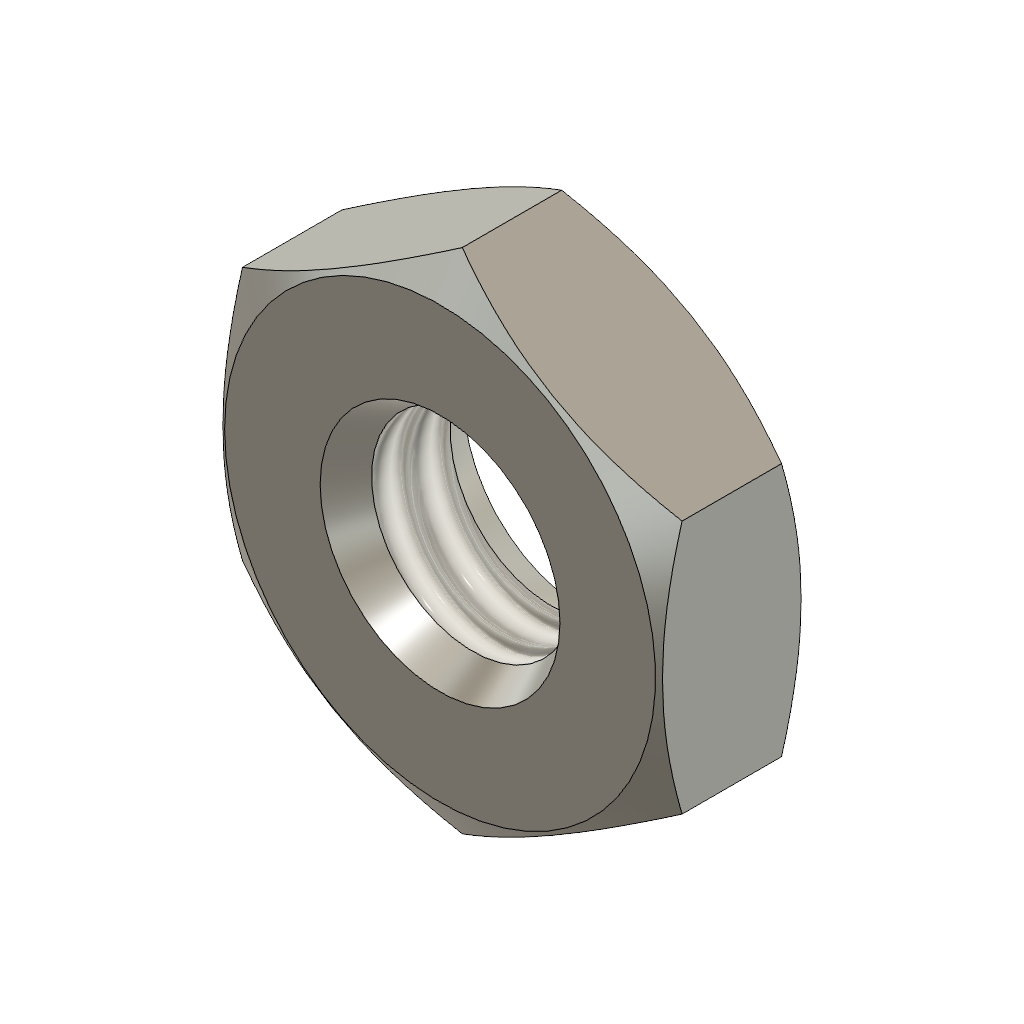
pencarriage (Autodesk Fusion 360 archive; units mm, degrees)
design "Hexagon Thin Nut ISO 4035 - M3 Steel 6 Plain"
description: Hexagon Thin Nut ISO 4035 - M3
part number: ISO 4035 - M3 Steel 6 Plain
Autodesk Fusion 360 part; units mm, degrees
sketch "Sketch1" plane through (0, 0, 0) normal (0, 1, 0) x (1, 0, 0)
  line L0 (0, 0) -> (0, -1.8)
  line L1 (-1.5, 0) -> (-2.695, 0)
  line L2 (-2.695, 0) -> (-3.1763, -0.2778)
  line L3 (-3.1763, -0.2778) -> (-3.1763, -1.5222)
  line L4 (-3.1763, -1.5222) -> (-2.695, -1.8)
  line L5 (-2.695, -1.8) -> (-1.5, -1.8)
  line L6 (-1.5, -1.8) -> (-1.5, 0)
  dimension "d121" = 3
  dimension "d122" = 30
  dimension "d123" = 30
  dimension "d128" = 6.3525
  dimension "d172" = 5.39
  dimension "d179" = 1.8
  constraint vertical L0
  constraint coincident L0 L0.end
  constraint coincident origin L0
  constraint horizontal L1
  constraint coincident L0.start L1
  constraint coincident L0.start origin
  constraint coincident L0.end L5
  constraint vertical L1.end L4.end
  measures "d122" angle of L1 L2
  measures "d123" angle of L4 L5
  measures "d179" distance of L1 L5
revolve "Revolve1" add sketch "Sketch1" angle 360 about axis through (0, 0, 0) along (0, 0, 1)
sketch "Sketch8" plane through (0, 0, 1.8) normal (0, 0, 1) x (1, 0, 0)
  line L0 (-2.75, -1.5894) -> (-2.75, 1.5894)
  circle A0 centre (0, 0) radius 1.5
  circle A1 centre (0, 0) radius 3.1763
  dimension "d114" = 2.75
  constraint coincident L0.end A1
  constraint coincident L0.start A1
  constraint vertical L0
  measures "d114" distance of A0.centre L0
extrude "Extrude5" cut sketch "Sketch8" against normal blind 1.8 contours L0 A1 picked at (-2.8188, -0.3871)
pattern_circular "C-Pattern2" count 6 over 360 about axis through (0, 0, 1.75) along (0, 0, 1) of "Extrude5"
thread "Thread3" "ISO Metric profile 3.0 M3x0.5 M3x0.5 6H" major diameter 3.086 minor diameter 2.529 pitch 0.5 angle 60 resizes the face on face at (-1.4981, 0.0748, 1.2)
sketch "Sketch12" plane through (0, 0, 0) normal (0, 1, 0) x (1, 0, 0)
  line L0 (-1.5, 0) -> (0, 0)
  line L1 (-0.9804, -0.9) -> (-1.5, 0)
  line L2 (-1.5, -1.8) -> (0, -1.8)
  line L3 (-0.9804, -0.9) -> (-1.5, -1.8)
  line L4 (0, 0) -> (0, -1.8)
  dimension "d169" = 60
  dimension "d177" = 1.5
  dimension "d178" = 60
  constraint horizontal L0
  constraint coincident L1.start L3.start
  constraint vertical L0.start L2.start
  constraint coincident L2.end L4.end
  constraint coincident L0.end L4.start
  constraint perpendicular L2 L4
  measures "d169" angle of L2 L3
  measures "d177" distance of L0.start L4
  measures "d178" angle of L0 L1
revolve "Revolve3" cut sketch "Sketch12" angle 360 about axis through (0, 0, 1.75) along (0, 0, 1)
equation "adsk_nheig = 1.80 mm"
equation "adsk_maxdia = 6.3525 mm"
equation "adsk_nomdia = 3.00 mm"
equation "d89 = -adsk_nheig"
equation "adsk_waflat = 5.50 mm"
equation "d114 = adsk_waflat / 2"
equation "adsk_chamang1 = 30.00 deg"
equation "adsk_chamang2 = 30.00 deg"
equation "d121 = adsk_nomdia"
equation "d122 = adsk_chamang1"
equation "d123 = adsk_chamang2"
equation "d128 = adsk_maxdia"
equation "d163 = adsk_nheig"
equation "adsk_beardia = 5.39 mm"
equation "d172 = adsk_beardia"
equation "d177 = adsk_nomdia * 0.5"
equation "d179 = adsk_nheig"

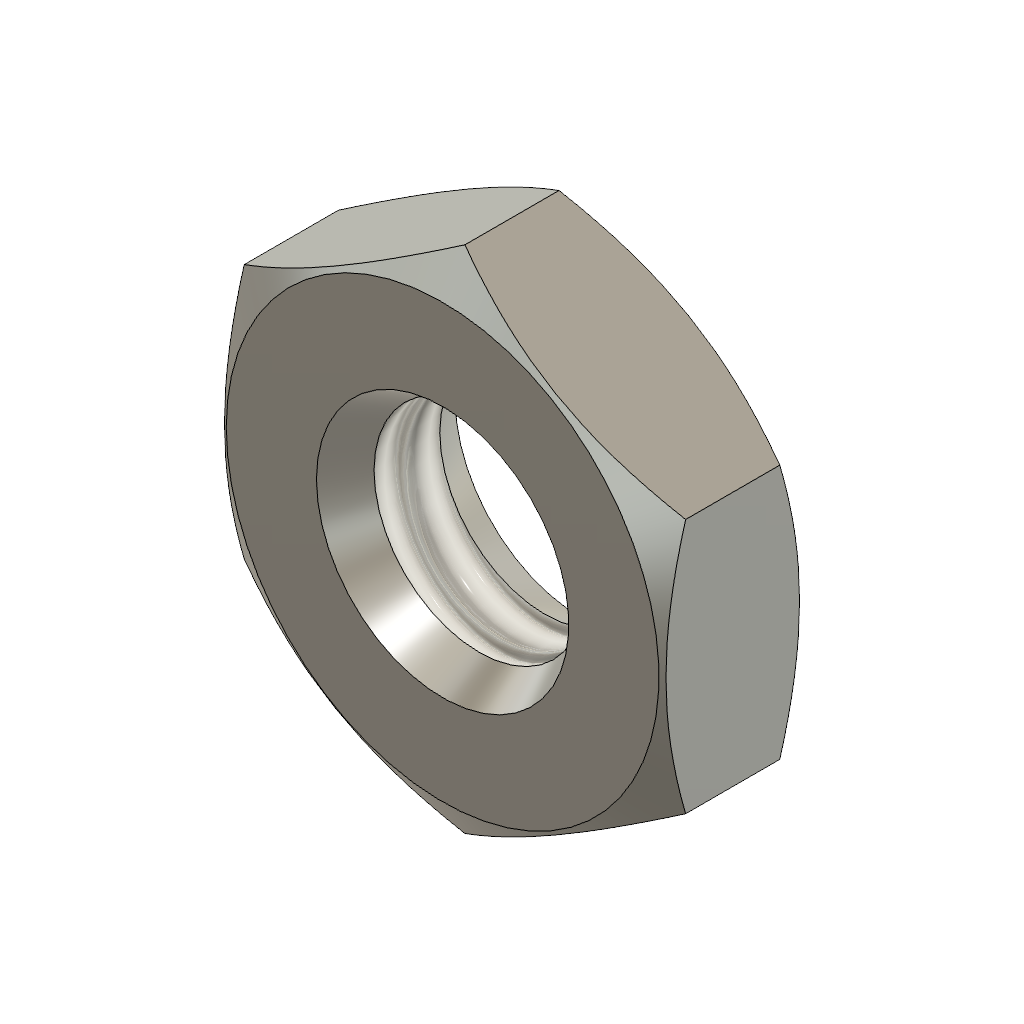
design "Hexagon Thin Nut ISO 4035 - M4 Steel 6 Plain"
description: Hexagon Thin Nut ISO 4035 - M4
part number: ISO 4035 - M4 Steel 6 Plain
Autodesk Fusion 360 part; units mm, degrees
sketch "Sketch1" plane through (0, 0, 0) normal (0, 1, 0) x (1, 0, 0)
  line L0 (0, 0) -> (0, -2.2)
  line L1 (-2, 0) -> (-3.43, 0)
  line L2 (-3.43, 0) -> (-4.0425, -0.3536)
  line L3 (-4.0425, -0.3536) -> (-4.0425, -1.8464)
  line L4 (-4.0425, -1.8464) -> (-3.43, -2.2)
  line L5 (-3.43, -2.2) -> (-2, -2.2)
  line L6 (-2, -2.2) -> (-2, 0)
  dimension "d121" = 4
  dimension "d122" = 30
  dimension "d123" = 30
  dimension "d128" = 8.085
  dimension "d172" = 6.86
  dimension "d179" = 2.2
  constraint vertical L0
  constraint coincident L0 L0.end
  constraint coincident origin L0
  constraint horizontal L1
  constraint coincident L0.start L1
  constraint coincident L0.start origin
  constraint coincident L0.end L5
  constraint vertical L1.end L4.end
  measures "d122" angle of L1 L2
  measures "d123" angle of L4 L5
  measures "d179" distance of L1 L5
revolve "Revolve1" add sketch "Sketch1" angle 360 about axis through (0, 0, 0) along (0, 0, 1)
sketch "Sketch8" plane through (0, 0, 2.2) normal (0, 0, 1) x (1, 0, 0)
  line L0 (-3.5, -2.0228) -> (-3.5, 2.0228)
  circle A0 centre (0, 0) radius 2
  circle A1 centre (0, 0) radius 4.0425
  dimension "d114" = 3.5
  constraint coincident L0.end A1
  constraint coincident L0.start A1
  constraint vertical L0
  measures "d114" distance of A0.centre L0
extrude "Extrude5" cut sketch "Sketch8" against normal blind 2.2 contours L0 A1 picked at (-3.5875, 0.4927)
pattern_circular "C-Pattern2" count 6 over 360 about axis through (0, 0, 1.75) along (0, 0, 1) of "Extrude5"
thread "Thread3" "ISO Metric profile 4.0 M4x0.7 M4x0.7 6H" major diameter 4.1095 minor diameter 3.332 pitch 0.7 angle 60 resizes the face on face at (-1.9975, 0.0997, 1.4667)
sketch "Sketch12" plane through (0, 0, 0) normal (0, 1, 0) x (1, 0, 0)
  line L0 (-2, 0) -> (0, 0)
  line L1 (-1.3649, -1.1) -> (-2, 0)
  line L2 (-2, -2.2) -> (0, -2.2)
  line L3 (-1.3649, -1.1) -> (-2, -2.2)
  line L4 (0, 0) -> (0, -2.2)
  dimension "d169" = 60
  dimension "d177" = 2
  dimension "d178" = 60
  constraint horizontal L0
  constraint coincident L1.start L3.start
  constraint vertical L0.start L2.start
  constraint coincident L2.end L4.end
  constraint coincident L0.end L4.start
  constraint perpendicular L2 L4
  measures "d169" angle of L2 L3
  measures "d177" distance of L0.start L4
  measures "d178" angle of L0 L1
revolve "Revolve3" cut sketch "Sketch12" angle 360 about axis through (0, 0, 1.75) along (0, 0, 1)
equation "adsk_nheig = 2.20 mm"
equation "adsk_maxdia = 8.085 mm"
equation "adsk_nomdia = 4.00 mm"
equation "d89 = -adsk_nheig"
equation "adsk_waflat = 7.00 mm"
equation "d114 = adsk_waflat / 2"
equation "adsk_chamang1 = 30.00 deg"
equation "adsk_chamang2 = 30.00 deg"
equation "d121 = adsk_nomdia"
equation "d122 = adsk_chamang1"
equation "d123 = adsk_chamang2"
equation "d128 = adsk_maxdia"
equation "d163 = adsk_nheig"
equation "adsk_beardia = 6.86 mm"
equation "d172 = adsk_beardia"
equation "d177 = adsk_nomdia * 0.5"
equation "d179 = adsk_nheig"

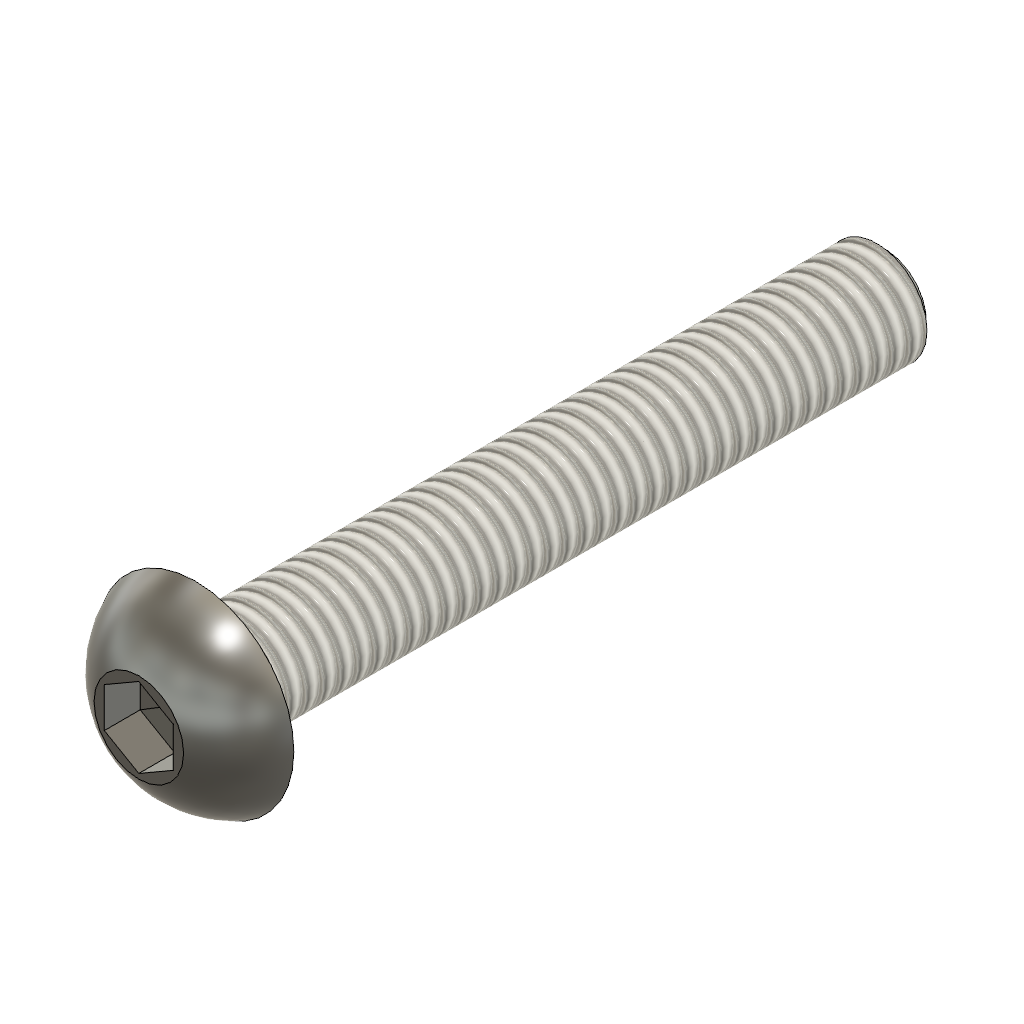
design "Forged Hexagon Socket Button Head Cap Screw ASME B18.3.4M - M3 x 0.5 x 20 Steel Grade 2 Plain"
description: Forged Hexagon Socket Button Head Cap Screw ASME B18.3.4M - M3 x 0.5 x 20
part number: FHSBHCS ASME B18.3.4M - M3 x 0.5 x 20 Steel Grade 2 Plain
Autodesk Fusion 360 part; units mm, degrees
sketch "Sketch1" plane through (0, 0, 0) normal (0, 1, 0) x (1, 0, 0)
  line L0 (-1.5, 0) -> (-1.5, 20)
  line L1 (-1.5, 20) -> (0, 20)
  line L2 (0, 20) -> (0, -1.65)
  line L3 (-1.5, 0) -> (-2.85, 0)
  line L4 (0, -1.65) -> (-1.3, -1.65)
  arc A0 (-2.85, 0) -> (-1.3, -1.65) centre (0, 1.1242) ccw
  dimension "d9" = 3
  dimension "d66" = 5.7
  dimension "d98" = 2.6
  dimension "d105" = 1.65
  dimension "d106" = 20
  constraint perpendicular L0 L1
  constraint perpendicular L0 L3
  constraint coincident origin L3
  constraint vertical L0
  constraint vertical L2
  constraint coincident origin L2
  constraint perpendicular L2 L4
  constraint coincident L2 A0.centre
  measures "d105" distance of L3 L4
  measures "d106" distance of origin L1
revolve "Revolve1" add sketch "Sketch1" angle 360 about axis through (0, 0, -20) along (0, 0, 1)
ref_plane "WorkPlane1" through (0, 0, 1.65) normal (0, 0, 1) x (1, 0, 0)
sketch "Sketch6" plane through (0, 0, 1.65) normal (0, 0, 1) x (1, 0, 0)
  line L0 (0, -1.1547) -> (1, -0.5774)
  line L1 (1, -0.5774) -> (1, 0.5774)
  line L2 (1, 0.5774) -> (0, 1.1547)
  line L3 (0, 1.1547) -> (-1, 0.5774)
  line L4 (-1, 0.5774) -> (-1, -0.5774)
  line L5 (-1, -0.5774) -> (0, -1.1547)
  dimension "d117" = 2
  constraint vertical L1
  measures "d117" distance of L1 L4
extrude "Extrude1" cut sketch "Sketch6" against normal blind 1.04
extrude "Extrude2" cut 1 faces at (-0.3333, -0.1925, 0.61) along direction (0, 0, -1) blind 1.04 draft -85
fillet "Fillet5" radius 0.1 1 edges at (-1.3985, 0.5424, 0)
thread "Thread5" "ANSI Metric M Profile 3.0 M3x0.5 M3x0.5 4g6g" major diameter 2.927 minor diameter 2.369 pitch 0.5 angle 60 resizes the face on face at (-1.4925, 0.1494, -6.7333) from (0, 0, -1) to (0, 0, -20)
sketch "Sketch5" plane through (0, 0, 0) normal (0, 1, 0) x (1, 0, 0)
  line L0 (0, 20) -> (0, -1.65)
  line L1 (0, 20) -> (-1.53, 20)
  line L2 (-1.53, 20) -> (-1.53, 19.6933)
  line L3 (-1.53, 19.6933) -> (-1.1933, 20)
  dimension "d108" = 0.3067
  dimension "d109" = 1.1933
  dimension "d110" = 1.53
  constraint coincident L0.start L1.start
  constraint perpendicular L1 L2
  constraint coincident L1 L3.end
  measures "d108" distance of L1 L2.end
  measures "d109" distance of L0 L3.end
  measures "d110" distance of L0 L2
revolve "Revolve2" cut sketch "Sketch5" angle 360 about axis through (0, 0, -20) along (0, 0, 1)
equation "d9 = adsk_nomdia"
equation "adsk_nomlen = 20.00 mm"
equation "adsk_headh = 1.65 mm"
equation "adsk_headdia = 5.70 mm"
equation "adsk_nomdia = 3.00 mm"
equation "adsk_philwidth = 2.00 mm"
equation "d31 = -adsk_phildepth"
equation "adsk_phildepth = 1.04 mm"
equation "d66 = adsk_headdia"
equation "d71 = adsk_headh"
equation "d76 = -adsk_phildepth"
equation "adsk_thrlen = 19.00 mm"
equation "adsk_endpointdia = 2.38655 mm"
equation "adsk_startlen = 0.306725 mm"
equation "d98 = adsk_philwidth * 1.3"
equation "adsk_midfillet = 0.10 mm"
equation "d104 = adsk_midfillet"
equation "d105 = adsk_headh"
equation "d106 = adsk_nomlen"
equation "d108 = adsk_startlen"
equation "d109 = adsk_endpointdia / 2"
equation "d110 = adsk_nomdia * 0.51"
equation "d116 = min(adsk_thrlen; adsk_nomlen - adsk_midfillet - 0.001 mm)"
equation "d117 = adsk_philwidth"
